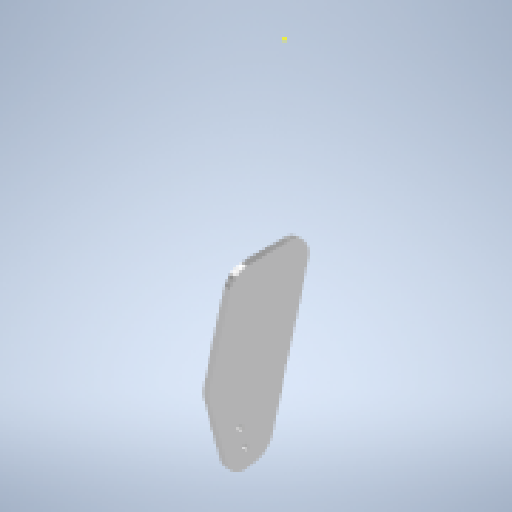
# Autodesk Inventor part: hand
Saved by Autodesk Inventor 2024.1 (Build 281209000, 209)
## iProperties
Created: 2024-02-14
Part Number: hand
Material: アルミニウム 6061
Document SubType Name: Modeling
Designer: hibik
Density: 2.7 g/cm^3
Appearance: アルミニウム - フラット
Author: hibik
Autodesk Inventor part; units mm, degrees
ref_plane "YZ Plane" through (0, 0, 0) normal (1, 0, 0) x (0, 1, 0)
ref_plane "XZ Plane" through (0, 0, 0) normal (0, 1, 0) x (-1, 0, 0)
ref_plane "XY Plane" through (0, 0, 0) normal (0, 0, 1) x (1, 0, 0)
sketch "スケッチ1" plane through (0, 0, 0) normal (1, 0, 0) x (0, 1, 0)
  circle A0 centre (0, 0) radius 13
  circle A1 centre (0, 0) radius 4.25
  circle A2 centre (0, 0) radius 6 construction
  circle A3 centre (6, 0) radius 1
  circle A4 centre (3, 5.1962) radius 1
  circle A5 centre (-3, 5.1962) radius 1
  circle A6 centre (-6, 0) radius 1
  circle A7 centre (-3, -5.1962) radius 1
  circle A8 centre (3, -5.1962) radius 1
  line L0 (0, 13) -> (-44.9356, 13)
  line L1 (-44.9356, 13) -> (-44.9356, -13)
  line L2 (-44.9356, -13) -> (0, -13)
  line L3 (0, -13) -> (0, 13)
  line L4 (-20, 6.3185) -> (-25.1764, -13)
  line L5 (-25.1764, -13) -> (-92.7912, 5.1173)
  line L6 (-92.7912, 5.1173) -> (-87.6148, 24.4358)
  line L7 (-87.6148, 24.4358) -> (-20, 6.3185)
  line L8 (-68.643, 19.3524) -> (-90.5498, 13.4825)
  line L9 (-87.9616, 3.8232) -> (-90.5498, 13.4825)
  circle A9 centre (-72.0415, 13.3611) radius 2.5
  circle A10 centre (-60.509, 10.271) radius 2.5
  circle A11 centre (-79.5332, 8.4667) radius 2.5
  circle A12 centre (-68.0007, 5.3766) radius 2.5
  circle A13 centre (-56.4682, 2.2864) radius 2.5
  line L10 (-72.0415, 13.3611) -> (-60.509, 10.271) construction
  line L11 (-79.5332, 8.4667) -> (-56.4682, 2.2864) construction
  line L12 (-72.0415, 13.3611) -> (-72.6885, 10.9463) construction
  line L13 (-79.5332, 8.4667) -> (-80.1803, 6.0519) construction
  line L14 (-68.0007, 5.3766) -> (-68.6477, 2.9618) construction
  line L15 (-79.5332, 8.4667) -> (-89.9539, 11.2589) construction
  line L16 (-56.4682, 2.2864) -> (-44.9356, -0.8037) construction
  line L17 (-56.4682, 2.2864) -> (-57.1152, -0.1284)
  point P0 (-3.3656, 12.5568)
  point P1 (-44.9356, -7.7055)
  dimension "d2" = 26
  dimension "d4" = 12
  dimension "d27" = 5
  dimension "d29" = 5
  dimension "d30" = 5
  dimension "d31" = 5
  dimension "d3" = 8.5
  dimension "d5" = 2
  dimension "d8" = 360
  dimension "d12" = 15
  dimension "d13" = 20
  dimension "d14" = 70
  dimension "d15" = 20
  dimension "d18" = 10
  dimension "d19" = 30
  dimension "d28" = 5
  dimension "d32" = 11.9393
  dimension "d33" = 11.9393
  dimension "d34" = 11.9393
  dimension "d35" = 5.9697
  dimension "d36" = 6.6667
  dimension "d37" = 6.6667
  dimension "d38" = 6.6667
  dimension "d39" = 11.9393
  dimension "d40" = 11.9393
  constraints: 36 end point, 8 centre point, 8 point on line, 7 perpendicular, 6 parallel, 3 coincident, 2 horizontal, 2 horizontal alignment, 2 midpoint, 1 collinear, 30 other
  measures "d3" diameter of A1
  measures "d5" diameter of A3
  measures "d12" angle of L0 L7
  measures "d13" distance from line of L4.start L3
  measures "d14" distance between parallel lines of L6 L4
  measures "d15" distance between parallel lines of L5 L7
  measures "d18" distance from line of L9.start L8
  measures "d19" angle of L7 L8
  measures "d28" diameter of A10
  measures "d32" distance from line of L10.end L12
  measures "d33" distance from line of L14.start L13
  measures "d34" distance from line of L11.end L14
  measures "d35" distance from line of L10.start L13
  measures "d36" distance between parallel lines of L7 L10
  measures "d37" distance between parallel lines of L11 L10
  measures "d38" distance between parallel lines of L5 L11
  measures "d39" distance from line of L11.start L6
  measures "d40" distance from line of L16.end L17
extrude "押し出し1" add sketch "スケッチ1" along normal blind 1.5 contours L1 L5 L9 L8 L7 | A9 | A10 | A11 | A12 | A13
fillet "フィレット1" radius 5 5 edges at (0.75, -68.643, 19.3524) (0.75, -90.5498, 13.4825) (0.75, -87.9616, 3.8232) (0.75, -44.9356, -7.7055) (0.75, -44.9356, 13)
sketch "スケッチ3" plane through (1.5, 0, 0) normal (1, 0, 0) x (0, 0, -1)
  point P0 (0, 0)
sketch "スケッチ4" plane through (1.5, 0, 0) normal (1, 0, 0) x (0, 0, -1)
  circle A0 centre (-9.947, -84.426) radius 0.8 projected
  circle A1 centre (-11.2411, -79.5964) radius 0.8 projected
  point P0 (0, 0)
extrude "押し出し2" cut sketch "スケッチ4" against normal through all
equation "\"d32\" = d40"
equation "\"d33\" = d32"
equation "\"d34\" = d33"
equation "\"d35\" = 0.5 * d33"
equation "\"d36\" = d38"
equation "\"d37\" = d38"
equation "\"d39\" = d40"
